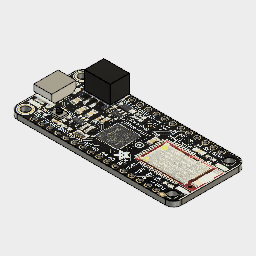
Generic Feather with Holes (Autodesk Fusion 360 design; units mm, degrees)
Autodesk Fusion 360 part; units mm, degrees
sketch "pcb" plane through (0, 0, 0) normal (0, 0, 1) x (1, 0, 0)
  line L0 (0, 0) -> (51.2, 0)
  line L1 (51.2, 0) -> (51.2, 22.8)
  line L2 (51.2, 22.8) -> (0, 22.8)
  line L3 (0, 22.8) -> (0, 0)
  circle A0 centre (2.54, 2.54) radius 1.25
  circle A1 centre (2.54, 20.32) radius 1.25
  circle A2 centre (48.26, 20.32) radius 1.25
  circle A3 centre (48.26, 2.54) radius 1.25
  line L4 (0, 11.4) -> (51.2, 11.4) construction
  line L5 (25.6, 22.8) -> (25.6, 0) construction
  line L6 (0, 1.27) -> (51.2, 1.27) construction
  circle A4 centre (24.33, 1.27) radius 0.635
  circle A5 centre (21.79, 1.27) radius 0.635
  circle A6 centre (19.25, 1.27) radius 0.635
  circle A7 centre (16.71, 1.27) radius 0.635
  circle A8 centre (14.17, 1.27) radius 0.635
  circle A9 centre (11.63, 1.27) radius 0.635
  circle A10 centre (9.09, 1.3) radius 0.635
  circle A11 centre (6.55, 1.27) radius 0.635
  circle A12 centre (26.87, 1.27) radius 0.635
  circle A13 centre (29.41, 1.27) radius 0.635
  circle A14 centre (31.95, 1.27) radius 0.635
  circle A15 centre (34.49, 1.27) radius 0.635
  circle A16 centre (39.57, 1.27) radius 0.635
  circle A17 centre (37.03, 1.27) radius 0.635
  circle A18 centre (42.11, 1.27) radius 0.635
  circle A19 centre (44.65, 1.27) radius 0.635
  circle A20 centre (44.65, 21.53) radius 0.635
  circle A21 centre (39.57, 21.53) radius 0.635
  circle A22 centre (34.49, 21.53) radius 0.635
  circle A23 centre (31.95, 21.53) radius 0.635
  circle A24 centre (29.41, 21.53) radius 0.635
  circle A25 centre (26.87, 21.53) radius 0.635
  circle A26 centre (42.11, 21.53) radius 0.635
  circle A27 centre (37.03, 21.53) radius 0.635
  circle A28 centre (24.33, 21.53) radius 0.635
  circle A29 centre (21.79, 21.53) radius 0.635
  circle A30 centre (19.25, 21.53) radius 0.635
  circle A31 centre (16.71, 21.53) radius 0.635
  dimension "d1" = 51.2
  dimension "d2" = 22.8
  dimension "d3" = 2.5
  dimension "d4" = 2.54
  dimension "d5" = 2.54
  dimension "d6" = 2.5
  dimension "d7" = 2.54
  dimension "d8" = 20.32
  dimension "d9" = 2.5
  dimension "d10" = 48.26
  dimension "d11" = 20.32
  dimension "d12" = 2.5
  dimension "d13" = 2.54
  dimension "d14" = 48.26
  dimension "d40" = 1.27
  dimension "d41" = 1.27
  dimension "d42" = 1.27
  dimension "d43" = 1.27
  dimension "d44" = 1.27
  dimension "d45" = 1.27
  dimension "d46" = 1.27
  dimension "d47" = 2.54
  dimension "d48" = 2.54
  dimension "d49" = 2.54
  dimension "d50" = 2.54
  dimension "d51" = 1.27
  dimension "d52" = 1.27
  dimension "d53" = 1.27
  dimension "d55" = 2.54
  dimension "d56" = 2.54
  dimension "d57" = 2.54
  dimension "d58" = 1.27
  dimension "d59" = 1.27
  dimension "d60" = 1.27
  dimension "d61" = 1.27
  dimension "d62" = 2.54
  dimension "d63" = 2.54
  dimension "d64" = 2.54
  dimension "d65" = 1.27
  dimension "d68" = 1.27
  dimension "d74" = 1.27
  dimension "d75" = 2.54
  dimension "d76" = 2.54
  dimension "d77" = 1.27
  dimension "d78" = 1.27
  dimension "d79" = 2.54
  dimension "d80" = 2.54
  measures "d1" distance of L1.end L2.end
  measures "d2" distance of L0.end L1.end
  measures "d3" diameter of A0
  measures "d4" distance of L3 A0.centre
  measures "d5" distance of L0 A0.centre
  measures "d6" diameter of A1
  measures "d7" distance of L3 A1.centre
  measures "d8" distance of L0 A1.centre
  measures "d9" diameter of A2
  measures "d10" distance of L3 A2.centre
  measures "d11" distance of L0 A2.centre
  measures "d12" diameter of A3
  measures "d13" distance of L0 A3.centre
  measures "d14" distance of L3 A3.centre
  measures "d40" distance of L0 L6
  measures "d41" diameter of A4
  measures "d42" distance of L5 A4.centre
  measures "d43" diameter of A5
  measures "d44" diameter of A6
  measures "d45" diameter of A7
  measures "d46" diameter of A8
  measures "d47" distance of A4.centre A5.centre
  measures "d48" distance of A5.centre A6.centre
  measures "d49" distance of A6.centre A7.centre
  measures "d50" distance of A7.centre A8.centre
  measures "d51" diameter of A9
  measures "d52" diameter of A10
  measures "d53" diameter of A11
  measures "d55" distance of A8.centre A9.centre
  measures "d56" distance of A9.centre A10.centre
  measures "d57" distance of A10.centre A11.centre
  measures "d58" diameter of A12
  measures "d59" diameter of A13
  measures "d60" diameter of A14
  measures "d61" diameter of A15
  measures "d62" distance of A14.centre A15.centre
  measures "d63" distance of A13.centre A14.centre
  measures "d64" distance of A12.centre A13.centre
  measures "d65" distance of L5 A12.centre
  measures "d68" diameter of A16
  measures "d74" diameter of A17
  measures "d75" distance of A15.centre A17.centre
  measures "d76" distance of A16.centre A17.centre
  measures "d77" diameter of A18
  measures "d78" diameter of A19
  measures "d79" distance of A16.centre A18.centre
  measures "d80" distance of A18.centre A19.centre
extrude "Extrude1" add sketch "pcb" against normal blind 1.6 makes body 1
fillet "Fillet1" radius 2.54 4 edges at (0, 0, -0.8) (0, 22.8, -0.8) (51.2, 0, -0.8) (51.2, 22.8, -0.8) on bodies 1
sketch "microusb" plane through (0, 0, 0) normal (0, 0, 1) x (-1, 0, 0)
  arc A0 (-51.2, -20.26) -> (-48.66, -22.8) centre (-48.66, -20.26) ccw
  line L0 (-48.66, -22.8) -> (-2.54, -22.8)
  arc A1 (-2.54, -22.8) -> (0, -20.26) centre (-2.54, -20.26) ccw
  line L1 (0, -20.26) -> (0, -2.54)
  arc A2 (0, -2.54) -> (-2.54, 0) centre (-2.54, -2.54) ccw
  line L2 (-2.54, 0) -> (-48.66, 0)
  arc A3 (-48.66, 0) -> (-51.2, -2.54) centre (-48.66, -2.54) ccw
  line L3 (-51.2, -2.54) -> (-51.2, -20.26)
  circle A4 centre (-2.54, -2.54) radius 1.25
  circle A5 centre (-48.26, -20.32) radius 1.25
  circle A6 centre (-48.26, -2.54) radius 1.25
  circle A7 centre (-2.54, -20.32) radius 1.25
  line L4 (0, -15.23) -> (-5.6, -15.23)
  line L5 (-5.6, -15.23) -> (-5.6, -7.63)
  line L6 (-5.6, -7.63) -> (0, -7.63)
  line L7 (0, -7.63) -> (0, -15.23)
  line L8 (-5.6, -11.43) -> (0, -11.43) construction
  circle A8 centre (-11.63, -1.27) radius 0.635
  circle A9 centre (-9.09, -1.3) radius 0.635
  circle A10 centre (-6.55, -1.27) radius 0.635
  circle A11 centre (-14.17, -1.27) radius 0.635
  circle A12 centre (-24.33, -1.27) radius 0.635
  circle A13 centre (-21.79, -1.27) radius 0.635
  circle A14 centre (-19.25, -1.27) radius 0.635
  circle A15 centre (-16.71, -1.27) radius 0.635
  circle A16 centre (-16.71, -21.53) radius 0.635
  circle A17 centre (-31.95, -21.53) radius 0.635
  circle A18 centre (-19.25, -21.53) radius 0.635
  circle A19 centre (-21.79, -21.53) radius 0.635
  circle A20 centre (-42.11, -21.53) radius 0.635
  circle A21 centre (-29.41, -21.53) radius 0.635
  circle A22 centre (-26.87, -21.53) radius 0.635
  circle A23 centre (-37.03, -21.53) radius 0.635
  circle A24 centre (-24.33, -21.53) radius 0.635
  circle A25 centre (-31.95, -1.27) radius 0.635
  circle A26 centre (-34.49, -1.27) radius 0.635
  circle A27 centre (-39.57, -1.27) radius 0.635
  circle A28 centre (-37.03, -1.27) radius 0.635
  circle A29 centre (-42.11, -1.27) radius 0.635
  circle A30 centre (-44.65, -1.27) radius 0.635
  circle A31 centre (-44.65, -21.53) radius 0.635
  circle A32 centre (-39.57, -21.53) radius 0.635
  circle A33 centre (-34.49, -21.53) radius 0.635
  circle A34 centre (-29.41, -1.27) radius 0.635
  circle A35 centre (-26.87, -1.27) radius 0.635
  dimension "d18" = 7.6
  dimension "d19" = 5.6
  dimension "d20" = 11.43
  measures "d18" distance of L4.end L5.end
  measures "d19" distance of L4.start L4.end
  measures "d20" distance of L2 L8
extrude "Extrude2" add sketch "microusb" along normal blind 2.95 separate body contours L1 L4 L5 L6 L7 makes body 2
chamfer "Chamfer1" distance 1 angle 45 2 edges at (2.8, 15.23, 0) (2.8, 7.63, 0) on bodies 2
sketch "jst" plane through (0, 0, 0) normal (0, 0, 1) x (-1, 0, 0)
  arc A0 (-51.2, -20.26) -> (-48.66, -22.8) centre (-48.66, -20.26) ccw
  line L0 (-48.66, -22.8) -> (-2.54, -22.8)
  arc A1 (-2.54, -22.8) -> (0, -20.26) centre (-2.54, -20.26) ccw
  line L1 (0, -20.26) -> (0, -2.54)
  arc A2 (0, -2.54) -> (-2.54, 0) centre (-2.54, -2.54) ccw
  line L2 (-2.54, 0) -> (-48.66, 0)
  arc A3 (-48.66, 0) -> (-51.2, -2.54) centre (-48.66, -2.54) ccw
  line L3 (-51.2, -2.54) -> (-51.2, -20.26)
  circle A4 centre (-2.54, -2.54) radius 1.25
  circle A5 centre (-48.26, -20.32) radius 1.25
  circle A6 centre (-48.26, -2.54) radius 1.25
  circle A7 centre (-2.54, -20.32) radius 1.25
  line L4 (-6.668, -22.8) -> (-14.668, -22.8)
  line L5 (-14.668, -22.8) -> (-14.668, -16.8)
  line L6 (-14.668, -16.8) -> (-6.668, -16.8)
  line L7 (-6.668, -16.8) -> (-6.668, -22.8)
  line L8 (-10.668, -22.8) -> (-10.668, -16.8) construction
  circle A8 centre (-11.63, -1.27) radius 0.635
  circle A9 centre (-9.09, -1.3) radius 0.635
  circle A10 centre (-6.55, -1.27) radius 0.635
  circle A11 centre (-14.17, -1.27) radius 0.635
  circle A12 centre (-24.33, -1.27) radius 0.635
  circle A13 centre (-21.79, -1.27) radius 0.635
  circle A14 centre (-19.25, -1.27) radius 0.635
  circle A15 centre (-16.71, -1.27) radius 0.635
  circle A16 centre (-16.71, -21.53) radius 0.635
  circle A17 centre (-31.95, -21.53) radius 0.635
  circle A18 centre (-19.25, -21.53) radius 0.635
  circle A19 centre (-21.79, -21.53) radius 0.635
  circle A20 centre (-42.11, -21.53) radius 0.635
  circle A21 centre (-29.41, -21.53) radius 0.635
  circle A22 centre (-26.87, -21.53) radius 0.635
  circle A23 centre (-37.03, -21.53) radius 0.635
  circle A24 centre (-24.33, -21.53) radius 0.635
  circle A25 centre (-31.95, -1.27) radius 0.635
  circle A26 centre (-34.49, -1.27) radius 0.635
  circle A27 centre (-39.57, -1.27) radius 0.635
  circle A28 centre (-37.03, -1.27) radius 0.635
  circle A29 centre (-42.11, -1.27) radius 0.635
  circle A30 centre (-44.65, -1.27) radius 0.635
  circle A31 centre (-44.65, -21.53) radius 0.635
  circle A32 centre (-39.57, -21.53) radius 0.635
  circle A33 centre (-34.49, -21.53) radius 0.635
  circle A34 centre (-29.41, -1.27) radius 0.635
  circle A35 centre (-26.87, -1.27) radius 0.635
  dimension "d24" = 8
  dimension "d25" = 6
  dimension "d26" = 10.668
  measures "d24" distance of L4.start L4.end
  measures "d25" distance of L4.start L6.end
  measures "d26" distance of L1 L8
extrude "Extrude3" add sketch "jst" along normal blind 5.6 separate body contours L0 L4 L5 L6 L7 makes body 3
sketch "Reset" plane through (0, 0, 0) normal (0, 0, 1) x (-1, 0, 0)
  line L0 (-7.62, -5.08) -> (-10.82, -5.08)
  line L1 (-10.82, -5.08) -> (-10.82, -7.62)
  line L2 (-10.82, -7.62) -> (-7.62, -7.62)
  line L3 (-7.62, -7.62) -> (-7.62, -5.08)
  line L4 (-7.62, -5.08) -> (-10.82, -7.62) construction
  line L5 (-10.82, -5.08) -> (-7.62, -7.62) construction
  circle A0 centre (-9.22, -6.35) radius 0.75
  line L6 (0, -20.26) -> (0, -2.54)
  line L7 (-2.54, 0) -> (-48.66, 0)
  point P0 (-9.22, -6.35)
  dimension "d95" = 3.2
  dimension "d96" = 2.54
  dimension "d97" = 1.5
  dimension "d98" = 7.62
  dimension "d99" = 5.08
  measures "d95" distance of L1.end L2.end
  measures "d96" distance of L0.end L1.end
  measures "d97" diameter of A0
  measures "d98" distance of L3 L6
  measures "d99" distance of L0 L7
extrude "Extrude6" add sketch "Reset" along normal blind 0.5 separate body makes body 4
extrude "Extrude7" add sketch "Reset" along normal blind 1 separate body contours A0 makes body 5
sketch "jst pins" plane through (0, 22.8, 0) normal (0, 1, 0) x (-1, 0, 0)
  line L0 (-14.668, 0) -> (-6.668, 0)
  line L1 (-6.668, 0) -> (-6.668, 5.6)
  line L2 (-6.668, 5.6) -> (-14.668, 5.6)
  line L3 (-14.668, 5.6) -> (-14.668, 0)
  line L4 (-14.168, 5.1) -> (-14.168, 0.5)
  line L5 (-14.168, 0.5) -> (-7.168, 0.5)
  line L6 (-7.168, 0.5) -> (-7.168, 5.1)
  line L7 (-7.168, 5.1) -> (-14.168, 5.1)
  line L8 (-10.668, 5.1) -> (-10.668, 0.5) construction
  circle A0 centre (-12.668, 3.1) radius 0.635
  circle A1 centre (-8.668, 3.1) radius 0.635
  dimension "d108" = 0.5
  dimension "d109" = 1.27
  dimension "d110" = 2
  dimension "d111" = 2
  measures "d109" diameter of A0
  measures "d110" distance of L8 A0.centre
  measures "d111" distance of L7 A0.centre
extrude "Extrude8" cut sketch "jst pins" against normal blind 1 contours L4 L5 L6 L7 bodies 3
equation "HoleDia = 1.27 mm"
equation "HoleSpace = 0.1 in"
equation "Hole2Edge = 0.05 in"
equation "d40 = Hole2Edge"
equation "d41 = HoleDia"
equation "d42 = HoleSpace / 2"
equation "d43 = HoleDia"
equation "d44 = HoleDia"
equation "d45 = HoleDia"
equation "d46 = HoleDia"
equation "d47 = HoleSpace"
equation "d48 = HoleSpace"
equation "d49 = HoleSpace"
equation "d50 = HoleSpace"
equation "d51 = HoleDia"
equation "d52 = HoleDia"
equation "d53 = HoleDia"
equation "d55 = HoleSpace"
equation "d56 = HoleSpace"
equation "d57 = HoleSpace"
equation "d58 = HoleDia"
equation "d59 = HoleDia"
equation "d60 = HoleDia"
equation "d61 = HoleDia"
equation "d62 = HoleSpace"
equation "d63 = HoleSpace"
equation "d64 = HoleSpace"
equation "d65 = HoleSpace / 2"
equation "d68 = HoleDia"
equation "d74 = HoleDia"
equation "d75 = HoleSpace"
equation "d76 = HoleSpace"
equation "d77 = HoleDia"
equation "d78 = HoleDia"
equation "d79 = HoleSpace"
equation "d80 = HoleSpace"
equation "PinLength = 10.6 mm"
equation "HoleDepth = 4.6 mm"
equation "d109 = HoleDia"
named bodies: "pcb", "usb", "jst", "Reset Switch"
